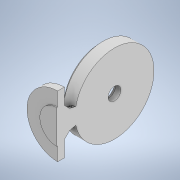
# Autodesk Inventor part: Part2
Saved by Autodesk Inventor 2020 (Build 240168000, 168)
## iProperties
Created: 2020-08-15
Part Number: Part2
Material: Generic
Document SubType Name: Modeling
Designer: benny
Density: 1 g/cm^3
Appearance: Default
Author: benny
Autodesk Inventor part; units mm, degrees
ref_plane "XZ Plane" through (0, 0, 0) normal (0, 1, 0) x (-1, 0, 0)
ref_plane "Work Plane1" through (0, 0, 0) normal (0, 0, 1) x (1, 0, 0)
sketch "Sketch1" plane through (0, 0, 0) normal (0, 0, 1) x (1, 0, 0)
  line L0 (0, -123) -> (-36, -123)
  line L1 (-36, -123) -> (-36, -115)
  line L2 (-36, -115) -> (-41.2, -115)
  line L3 (-41.2, -115) -> (-41.2, -112)
  line L4 (-41.2, -112) -> (-46, -112)
  line L5 (-46, -112) -> (-46, -85.5)
  line L6 (-46, -85.5) -> (-41.2, -85.5)
  line L7 (-41.2, -85.5) -> (-41.2, -82.5)
  line L8 (-41.2, -82.5) -> (-40.0184, -82.5)
  line L9 (-32.2077, -50.5) -> (-38.5735, -50.5)
  line L10 (-38.5735, -50.5) -> (-38.5735, -42.5)
  line L11 (-0.0735, -20) -> (-17.0735, -20)
  line L12 (-17.0735, -20) -> (-8.5309, -27.2194)
  line L13 (-38.5735, -42.5) -> (-30.0735, -42.5)
  line L14 (-30.0735, -42.5) -> (-30.0735, -39.5)
  line L15 (-30.0735, -42.5) -> (-30.0735, -39.5)
  line L16 (-30.0735, -39.5) -> (-28.5671, -40.4033)
  line L17 (-26.5599, -40.4322) -> (-8.8432, -30.4911)
  line L18 (-38.5735, -50.5) -> (-29.5735, -50.5)
  line L19 (-30.2813, -53.0374) -> (-38.092, -81.0374)
  line L20 (-0.0735, -20) -> (0, -20)
  line L21 (0, -20) -> (0, -123)
  arc A0 (-40.0184, -82.5) -> (-38.092, -81.0374) centre (-40.0184, -80.5) ccw
  arc A1 (-30.2813, -53.0374) -> (-32.2077, -50.5) centre (-32.2077, -52.5) ccw
  arc A2 (-28.5671, -40.4033) -> (-26.5599, -40.4322) centre (-27.5386, -38.688) ccw
  arc A3 (-8.8432, -30.4911) -> (-8.5309, -27.2194) centre (-9.8218, -28.7469) ccw
  line L22 (-55.2, 0) -> (9.2, 0) projected
  point P0 (0, 0)
  point P1 (-38.5, -82.5)
  point P2 (-30.0735, -50.5)
  dimension "d1" = 36
  dimension "d2" = 8
  dimension "d3" = 5.2
  dimension "d4" = 3
  dimension "d5" = 4.8
  dimension "d6" = 26.5
  dimension "d7" = 4.8
  dimension "d8" = 3
  dimension "d9" = 2.7
  dimension "d10" = 8.5
  dimension "d11" = 8
  dimension "d12" = 17
  dimension "d13" = 50.5
  dimension "d14" = 8.5
  dimension "d15" = 3
  dimension "d16" = 9
  dimension "d17" = 2
  constraints: 44 end point, 9 perpendicular, 8 point on circle, 8 tangent, 7 point on line, 5 horizontal, 4 centre point, 3 equal radius, 1 collinear
  measures "d1" distance of L0.start L0.end
  measures "d2" distance of L0.end L1.end
  measures "d3" distance of L1.end L2.end
  measures "d4" distance of L2.end L3.end
  measures "d5" distance of L3.end L4.end
  measures "d6" distance of L4.end L5.end
  measures "d7" distance of L5.end L6.end
  measures "d8" distance of L6.end L7.end
  measures "d9" distance of L7.end point (-38.5, -82.5)
  measures "d10" distance of point (-30.073, -50.5) L9.end
  measures "d11" distance of L9.end L10.end
  measures "d12" distance of L11.start L11.end
  measures "d13" distance from line of L9 point (0, 0)
  measures "d14" distance of L10.end L13.end
  measures "d15" distance of L13.end L14.end
  measures "d16" distance of L9.end L18.end
  measures "d17" radius of A0
revolve "Revolution1" add sketch "Sketch1" angle 360 about axis through (-10, 0, 0) along (1, 0, 0)
ref_plane "Work Plane2" through (0, 0, 0) normal (1, 0, 0) x (0, 1, 0)
sketch "Sketch2" plane through (0, 0, 0) normal (1, 0, 0) x (0, 1, 0)
  line L0 (0, 180) -> (52.5, 180)
  line L1 (52.5, 180) -> (52.5, 177)
  line L2 (52.5, 177) -> (55.5, 177)
  line L3 (55.5, 177) -> (95.5, 177)
  line L4 (95.5, 177) -> (95.5, 156)
  line L5 (95.5, 156) -> (46, 156)
  line L6 (46, 156) -> (34.2805, 144.2805)
  line L7 (46, 156) -> (81.8782, 156) construction
  line L8 (34.2805, 144.2805) -> (29.04, 139.04)
  line L9 (29.04, 139.04) -> (19.6091, 94.8986)
  line L10 (29.04, 139.04) -> (74.1776, 139.04) construction
  line L11 (19.6091, 94.8986) -> (0, 94.8986)
  line L12 (0, 94.8986) -> (0, 180)
  line L13 (29.04, 139.04) -> (29.6496, 137.8763)
  line L14 (29.6496, 137.8763) -> (28.7649, 133.7354)
  line L15 (28.7649, 133.7354) -> (27.7985, 133.2292)
  line L16 (27.761, 133.0538) -> (28.5818, 132.8784)
  line L17 (28.5818, 132.8784) -> (28.0079, 130.1923)
  line L18 (28.0079, 130.1923) -> (27.1871, 130.3677)
  line L19 (27.0764, 129.8494) -> (27.9346, 129.8494)
  line L20 (27.9346, 129.8494) -> (27.1871, 127.2568)
  line L21 (27.1871, 127.2568) -> (26.6395, 127.8044)
  line L22 (26.3419, 126.4116) -> (26.5379, 127.3288)
  line L23 (26.5303, 127.2934) -> (27.1343, 127.0736)
  line L24 (27.1343, 127.0736) -> (26.6909, 124.0283)
  line L25 (26.6909, 124.0283) -> (25.8586, 124.1495)
  line L26 (25.8235, 123.9853) -> (26.6801, 123.8023)
  line L27 (26.6801, 123.8023) -> (25.0618, 120.4197)
  circle A0 centre (0, 0) radius 123 projected
  line L28 (0, -183.6) -> (0, 240.6) projected
  point P0 (0, 123)
  dimension "d20" = 52.5
  dimension "d21" = 3
  dimension "d22" = 3
  dimension "d23" = 40
  dimension "d24" = 21
  dimension "d25" = 49.5
  dimension "d27" = 135
  dimension "d29" = 102.06
  constraints: 54 end point, 6 horizontal, 6 perpendicular, 5 point on line, 1 vertical, 18 other
  measures "d20" distance of L0.start L0.end
  measures "d21" distance of L0.end L1.end
  measures "d22" distance of L1.end L2.end
  measures "d23" distance of L2.end L3.end
  measures "d24" distance of L3.end L4.end
  measures "d25" distance of L4.end L5.end
  measures "d27" angle of L6 L7
revolve "Revolution2" add sketch "Sketch2" angle 180 about axis through (0, 0, -10) along (0, 0, 1) contours L0 L1 L2 L3 L4 L5 L6 L8 L9 A0 L12 | L9 L26 L27 | L9 L23 L24 L25 | L13 L14 L15 L9 | L9 L19 L20 L21 | L16 L17 L18 L9
body "Solid1"
